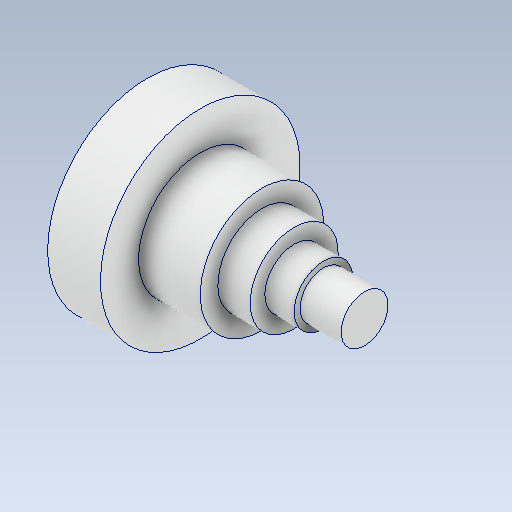
# Autodesk Inventor part: 5 Cilindros centrales
Saved by Autodesk Inventor 2021 (Build 250183000, 183)
## iProperties
Created: 2021-01-01
Part Number: 5 Cilindros centrales
Material: Aluminum 6061
Document SubType Name: Modeling
Designer: dieku
Density: 2.7 g/cm^3
Appearance: Aluminum - Flat
Author: dieku
Autodesk Inventor part; units mm, degrees
ref_plane "YZ Plane" through (0, 0, 0) normal (1, 0, 0) x (0, 1, 0)
ref_plane "XZ Plane" through (0, 0, 0) normal (0, 1, 0) x (-1, 0, 0)
ref_plane "XY Plane" through (0, 0, 0) normal (0, 0, 1) x (1, 0, 0)
sketch "Sketch1" plane through (0, 0, 0) normal (0, 0, 1) x (1, 0, 0)
  line L0 (0, 0) -> (0, 34)
  line L1 (0, 34) -> (18, 34)
  line L2 (18, 34) -> (18, 0)
  line L3 (18, 0) -> (18, 21)
  line L4 (18, 21) -> (39, 21)
  line L5 (39, 21) -> (39, 0)
  line L6 (39, 0) -> (39, 15)
  line L7 (39, 15) -> (50, 15)
  line L8 (50, 15) -> (50, 0)
  line L9 (50, 0) -> (50, 10)
  line L10 (50, 10) -> (60, 10)
  line L11 (60, 10) -> (60, 0)
  line L12 (60, 0) -> (60, 8)
  line L13 (60, 8) -> (74, 8)
  line L14 (74, 8) -> (74, 0)
  line L15 (0, 0) -> (74, 0)
  line L16 (0, 0) -> (84.2736, 0) construction
  dimension "d0" = 34
  dimension "d1" = 18
  dimension "d2" = 34
  dimension "d3" = 21
  dimension "d4" = 21
  dimension "d5" = 15
  dimension "d6" = 11
  dimension "d7" = 10
  dimension "d9" = 10
  dimension "d10" = 8
  dimension "d11" = 14
  constraints: 34 end point, 7 perpendicular, 4 point on line, 3 horizontal, 3 vertical
  measures "d0" distance of L0.start L0.end
  measures "d1" distance of L0.end L1.end
  measures "d2" distance of L1.end L2.end
  measures "d3" distance of L2.end L3.end
  measures "d4" distance of L3.end L4.end
  measures "d5" distance of L5.end L6.end
  measures "d6" distance of L6.end L7.end
  measures "d7" distance of L8.end L9.end
  measures "d9" distance of L9.end L10.end
  measures "d10" distance of L11.end L12.end
  measures "d11" distance of L12.end L13.end
revolve "Revolution1" add sketch "Sketch1" angle 360 about axis through (0, 0, 0) along (1, 0, 0)
body "Solid1"
